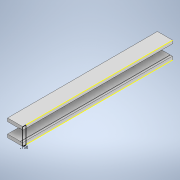
# Autodesk Inventor part: box slabs
Saved by Autodesk Inventor 2021 (Build 250183000, 183)
## iProperties
Created: 2021-07-05
Part Number: box slabs
Material: Generic
Document SubType Name: Modeling
Designer: newic
Density: 1 g/cm^3
Appearance: Default
Author: newic
Autodesk Inventor part; units mm, degrees
ref_plane "YZ Plane" through (0, 0, 0) normal (1, 0, 0) x (0, 1, 0)
ref_plane "XZ Plane" through (0, 0, 0) normal (0, 1, 0) x (-1, 0, 0)
ref_plane "XY Plane" through (0, 0, 0) normal (0, 0, 1) x (1, 0, 0)
sketch "Sketch1" plane through (0, 0, 0) normal (0, 0, 1) x (1, 0, 0)
  line L0 (0, 0) -> (88.9, 0)
  line L1 (88.9, 0) -> (88.9, 19.05)
  line L2 (88.9, 19.05) -> (0, 19.05)
  line L3 (0, 19.05) -> (0, 0)
  dimension "d0" = 88.9
  dimension "d1" = 19.05
  constraints: 8 end point, 2 parallel, 1 horizontal, 1 perpendicular
  measures "d0" distance of L2.end L1.end
  measures "d1" distance of L1.end L0.end
extrude "Extrusion1" add sketch "Sketch1" along normal blind 889
sketch "Sketch2" plane through (0, 19.05, 0) normal (0, 1, 0) x (1, 0, 0)
  line L0 (88.9, 0) -> (0, 0) projected
  line L1 (0, 0) -> (0, -889) projected
  line L2 (88.9, -889) -> (0, -889) projected
  line L3 (88.9, 0) -> (88.9, -889) projected
extrude "Extrusion2" add sketch "Sketch2" along normal blind 127
sketch "Sketch3" plane through (88.9, 0, 889) normal (1, 0, 0) x (0, 0, -1)
  line L0 (889, 0) -> (889, 146.05) projected
  line L1 (0, 146.05) -> (889, 146.05) projected
  line L2 (0, 0) -> (0, 146.05) projected
  line L3 (889, 0) -> (0, 0) projected
  line L4 (889, 0) -> (0, 0) projected
  line L5 (889, 0) -> (889, 146.05) projected
  line L6 (0, 0) -> (889, 0)
  line L7 (889, 0) -> (889, 19.05)
  line L8 (889, 19.05) -> (0, 19.05)
  line L9 (0, 19.05) -> (0, 0)
  line L10 (0, 0) -> (0, 146.05) projected
  line L11 (889, 0) -> (889, 146.05) projected
  line L12 (0, 0) -> (889, 0)
  line L13 (889, 0) -> (889, 101.6)
  line L14 (889, 101.6) -> (0, 101.6)
  line L15 (0, 101.6) -> (0, 0)
  line L16 (0, 101.6) -> (889, 101.6)
  line L17 (889, 101.6) -> (889, 82.55)
  line L18 (889, 82.55) -> (0, 82.55)
  line L19 (0, 82.55) -> (0, 101.6)
  dimension "d6" = 19.05
  dimension "d7" = 889
  dimension "d8" = 101.6
  dimension "d9" = 19.05
  constraints: 24 end point, 6 parallel, 3 horizontal, 3 perpendicular, 3 point on line
  measures "d6" distance of L7.end L6.end
  measures "d7" distance of L0.start L2.start
  measures "d8" distance of L13.end L12.end
  measures "d9" distance of L16.end L17.end
extrude "Extrusion3" cut sketch "Sketch3" against normal blind 127 contours L8 L2 L18 L0 | L14 L2 L1 L0
sketch "Sketch5" plane through (0, 0, 889) normal (0, 0, 1) x (1, 0, 0)
  line L0 (0, 0) -> (0, 19.05) projected
  line L1 (88.9, 82.55) -> (88.9, 101.6) projected
  line L2 (0, 0) -> (88.9, 0)
  line L3 (88.9, 0) -> (88.9, 101.6)
  line L4 (88.9, 101.6) -> (0, 101.6)
  line L5 (0, 101.6) -> (0, 0)
  line L6 (88.9, 19.05) -> (0, 19.05) projected
  line L7 (0, 82.55) -> (88.9, 82.55) projected
  line L8 (88.9, 82.55) -> (82.55, 82.55)
  line L9 (82.55, 82.55) -> (82.55, 74.8219)
  line L10 (82.55, 74.8219) -> (88.9, 74.8219)
  line L11 (88.9, 74.8219) -> (88.9, 82.55)
  line L12 (82.55, 82.55) -> (69.85, 82.55)
  line L13 (69.85, 82.55) -> (69.85, 85.725)
  line L14 (69.85, 85.725) -> (82.55, 85.725)
  line L15 (82.55, 85.725) -> (82.55, 82.55)
  dimension "d12" = 88.9
  dimension "d13" = 101.6
  dimension "d14" = 19.05
  dimension "d15" = 63.5
  dimension "d16" = 6.35
  dimension "d17" = 12.7
  dimension "d18" = 3.175
  constraints: 24 end point, 6 parallel, 3 horizontal, 3 perpendicular
  measures "d12" distance of L1.end L4.end
  measures "d13" distance of L2.end L1.end
  measures "d14" distance of L1.start L1.end
  measures "d15" distance between parallel lines of L6 L7
  measures "d16" distance of L10.end L9.end
  measures "d17" distance of L13.end L14.end
  measures "d18" distance of L12.end L13.end
extrude "Extrusion4" cut sketch "Sketch5" against normal through all contours L13 L14 L15 L7
sketch "Sketch6" plane through (0, 0, 889) normal (0, 0, 1) x (1, 0, 0)
  line L0 (0, 0) -> (0, 19.05)
  line L1 (88.9, 82.55) -> (88.9, 101.6)
  line L2 (0, 0) -> (88.9, 0)
  line L3 (88.9, 0) -> (88.9, 101.6)
  line L4 (88.9, 101.6) -> (0, 101.6)
  line L5 (0, 101.6) -> (0, 0)
  line L6 (88.9, 19.05) -> (0, 19.05)
  line L7 (0, 82.55) -> (88.9, 82.55)
  line L8 (88.9, 82.55) -> (82.55, 82.55)
  line L9 (82.55, 82.55) -> (82.55, 74.8219)
  line L10 (82.55, 74.8219) -> (88.9, 74.8219)
  line L11 (88.9, 74.8219) -> (88.9, 82.55)
  line L12 (82.55, 82.55) -> (69.85, 82.55)
  line L13 (69.85, 82.55) -> (69.85, 85.725)
  line L14 (69.85, 85.725) -> (82.55, 85.725)
  line L15 (82.55, 85.725) -> (82.55, 82.55)
  line L16 (76.2, 82.55) -> (76.2, 19.05)
  line L17 (88.9, 19.05) -> (0, 19.05) projected
  line L18 (76.2, 19.05) -> (76.2, 15.875)
  line L19 (76.2, 15.875) -> (72.9644, 24.7648)
  line L20 (76.2, 15.875) -> (79.0952, 23.8296)
  point P0 (75.0444, 19.05)
  point P1 (77.3556, 19.05)
  dimension "d21" = 88.9
  dimension "d22" = 101.6
  dimension "d23" = 19.05
  dimension "d24" = 63.5
  dimension "d25" = 6.35
  dimension "d26" = 12.7
  dimension "d27" = 3.175
  dimension "d28" = 3.175
  dimension "d29" = 20
  dimension "d30" = 20
  constraints: 40 end point, 6 parallel, 5 perpendicular, 3 horizontal, 1 midpoint, 1 point on line
  measures "d21" distance of L1.end L4.end
  measures "d22" distance of L2.end L1.end
  measures "d23" distance of L1.start L1.end
  measures "d24" distance between parallel lines of L6 L7
  measures "d25" distance of L10.end L9.end
  measures "d26" distance of L13.end L14.end
  measures "d27" distance of L12.end L13.end
  measures "d28" distance of L16.end L18.end
  measures "d29" angle of L19 L16
  measures "d30" angle of L20 L16
extrude "Extrusion5" cut sketch "Sketch6" against normal through all contours L6 L18 L19 | L6 L20 L18
sketch "Sketch8" plane through (88.9, 82.55, 889) normal (1, 0, 0) x (0, 0, -1)
  line L0 (889, 19.05) -> (0, 19.05) projected
  line L1 (889, -82.55) -> (0, -82.55) projected
  line L2 (0, 19.05) -> (19.05, 19.05)
  line L3 (19.05, 19.05) -> (19.05, -82.55)
  line L4 (19.05, -82.55) -> (0, -82.55)
  line L5 (0, -82.55) -> (0, 19.05)
  dimension "d40" = 19.05
  constraints: 8 end point, 2 parallel, 1 horizontal, 1 perpendicular, 1 point on line
  measures "d40" distance of L3.end L4.end
body "Solid1"
